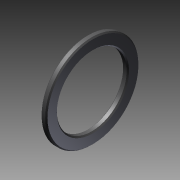
# Autodesk Inventor part: WSSS16-12-1
Saved by Autodesk Inventor 2011 SP1 (Build 150282100, 282)
## iProperties
Created: 2016-04-08
Part Number: WSSS16-12-1
Catalog Web Link: www.cadenas.de
Description: WSSB, WSSM, WSSS-Metal Washers - Standard Class - T Dimension Selectable -
Vendor: MISUMI
Document SubType Name: Modeling
Designer: psAdmin
Manufacturer: MISUMI
Mass: 0.084446 g
Surface Area: 2.43282 cm^2
Volume: 0.084446 cm^3
Density: 1 g/cm^3
Category: PARTsolutions
Company: MISUMI
Title: WSSS16-12-1
Author: Cadenas PARTsolutions
Comments: Metal Washers - Standard Class - T Dimension Selectable -
PSOL_IDENT_0: {$CADENAS_DATA\23d-libs\misumi\metric\26_washers_collars\wssb.prj},185 {VTYP=3D},{NB=WSSS16-12-1},{L
PSOL_IDENT_1: INA=WSSS16-12-1},{NN=WSSB, WSSM, WSSS},{DATE=10.11.2015 01:59:27},{GEOMDATE=06.10.2015 03:29:00},{VE
PSOL_IDENT_2: RSION=},{LINEID=290},{LINESUBID=-1},{WBVAR=MAT,ST,V,T}  {NB=WSSS16-12-1},{LINA=WSSS16-12-1},{KT=DUMM
PSOL_IDENT_3: Y},{PN=WSSS16-12-1},{TYPE=WSSS},{MAT=304},{ST=-},{STALG= '-','-' },{DALG=4,5,6,8,10,12,13,14,15,16,2
PSOL_IDENT_4: 0,25,30,35,40,50,60},{D=16},{V=12},{VALG=4,5,6,8,10,12},{T=1.0},{TALG=1,1.5,2,2.5,3,4,5,6,8},{C=0.2}
NN: WSSB, WSSM, WSSS
NT: Metal Washers - Standard Class - T Dimension Selectable -
NB: WSSS16-12-1
NBSYN: $PN.
LINA: WSSS16-12-1
PN: WSSS16-12-1
MAT: 304 Stainless Steel
ST: -
D: 16
V: 12
T: 1.0
SUPPLIER: MISUMI
ARTICLENO: WSSS16-12-1
BOMINFO: WSSS16-12-1
CREATOR: CADENAS GmbH
Autodesk Inventor part; units mm, degrees
sketch "Sketch_1" plane through (0, 0, 0) normal (0, 0, 1) x (1, 0, 0)
  line L0 (-3, 0) -> (3, 0)
  line L1 (0, -6.2) -> (0, -7.8)
  line L2 (0, -7.8) -> (0.2, -8)
  line L3 (0.2, -8) -> (0.8, -8)
  line L4 (0.8, -8) -> (1, -7.8)
  line L5 (1, -7.8) -> (1, -6.2)
  line L6 (1, -6.2) -> (0.8, -6)
  line L7 (0.8, -6) -> (0.2, -6)
  line L8 (0.2, -6) -> (0, -6.2)
  constraints: 18 end point
revolve "Revolution1" add sketch "Sketch_1" angle 360 about axis through (-3, 0, 0) along (-1, 0, 0)
ref_plane "a_XY" through (0, 0, 0) normal (1, 0, 0) x (0, 0, -1)
ref_plane "a_YZ" through (0, 0, 0) normal (0, 0, -1) x (0, 1, 0)
ref_plane "a_ZX" through (0, 0, 0) normal (0, 1, 0) x (1, 0, 0)
body "Solid1"
